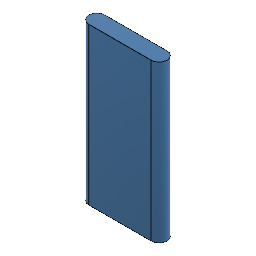
logger v4 (Autodesk Fusion 360 archive; units mm, degrees)
design "powerbank"
Autodesk Fusion 360 part; units mm, degrees
sketch "Sketch1" plane through (0, 0, 0) normal (0, 1, 0) x (1, 0, 0)
  line L0 (7.65, 0) -> (66.25, 0)
  line L1 (66.25, -15.3) -> (7.65, -15.3)
  arc A0 (7.65, 0) -> (7.65, -15.3) centre (7.65, -7.65) ccw
  arc A1 (66.25, -15.3) -> (66.25, 0) centre (66.25, -7.65) ccw
  constraint horizontal L0
  constraint horizontal L1
  constraint tangent L0 A0
  constraint tangent L1 A0
  constraint tangent L0 A1
  constraint tangent L1 A1
extrude "Extrude1" add sketch "Sketch1" along normal blind 147.8

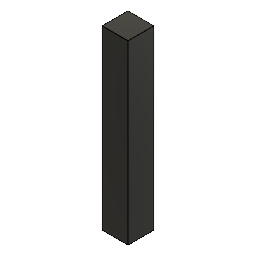
design "cable_margin"
Autodesk Fusion 360 part; units mm, degrees
sketch "Sketch1" plane through (0, 0, 0) normal (0, 1, 0) x (1, 0, 0)
  line L0 (0, 0) -> (2.5, 0)
  line L1 (2.5, 0) -> (2.5, -2.5)
  line L2 (2.5, -2.5) -> (0, -2.5)
  line L3 (0, -2.5) -> (0, 0)
  dimension "d1" = 2.5
  dimension "d2" = 2.5
  constraint horizontal L0
  constraint vertical L1
  constraint horizontal L2
  constraint vertical L3
  constraint coincident L0.start L3.end
  measures "d1" distance of L0.start L0.end
  measures "d2" distance of L0.start L2.end
extrude "Extrude1" add sketch "Sketch1" along normal blind 17
